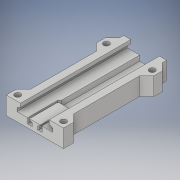
# Autodesk Inventor part: Holder_Mount
Saved by Autodesk Inventor 2019 (Build 230136000, 136)
## iProperties
Created: 2021-01-19
Part Number: Holder_Mount
Material: Generic
Document SubType Name: Modeling
Designer: zhanb
Density: 1 g/cm^3
Appearance: Default
Author: zhanb
Autodesk Inventor part; units mm, degrees
ref_plane "YZ Plane" through (0, 0, 0) normal (1, 0, 0) x (0, 1, 0)
ref_plane "XZ Plane" through (0, 0, 0) normal (0, 1, 0) x (-1, 0, 0)
ref_plane "XY Plane" through (0, 0, 0) normal (0, 0, 1) x (1, 0, 0)
sketch "Sketch1" plane through (0, 0, 0) normal (0, 1, 0) x (-1, 0, 0)
  line L0 (-25.4, 57.15) -> (25.4, 57.15)
  line L1 (25.4, 57.15) -> (25.4, -57.15)
  line L2 (25.4, -57.15) -> (-25.4, -57.15)
  line L3 (-25.4, -57.15) -> (-25.4, 57.15)
  line L4 (-25.4, 57.15) -> (25.4, -57.15) construction
  line L5 (25.4, 57.15) -> (-25.4, -57.15) construction
  point P0 (0, 0)
  dimension "d0" = 50.8
  dimension "d1" = 114.3
  constraints: 12 end point, 2 midpoint, 2 parallel, 1 horizontal, 1 perpendicular
  measures "d0" distance of L1.end L2.end
  measures "d1" distance of L2.end L0.start
extrude "Extrusion1" add sketch "Sketch1" along normal blind 15.875
ref_plane "Work Plane1" through (-25.4, 0, 31.75) normal (0, 0, 1) x (1, 0, 0)
sketch "Sketch2" plane through (-25.4, 0, 31.75) normal (0, 0, 1) x (1, 0, 0)
  line L0 (50.8, 0) -> (0, 0) construction
  line L1 (50.8, 0) -> (50.8, 15.875) construction
  line L2 (0, 15.875) -> (50.8, 15.875) construction
  line L3 (0, 0) -> (0, 15.875) construction
  line L4 (0, 15.875) -> (50.8, 15.875) construction
  line L5 (25.4, 15.875) -> (25.4, 0) construction
  line L6 (50.8, 0) -> (0, 0) construction
  line L7 (6.35, 15.875) -> (6.35, 0) construction
  circle A0 centre (25.4, 16.891) radius 5.08 construction
  line L8 (12.7, 15.875) -> (12.7, 12.7)
  line L9 (12.7, 12.7) -> (9.525, 10.8669)
  line L10 (9.525, 10.8669) -> (9.525, 7.9375)
  line L11 (9.525, 7.9375) -> (19.05, 7.9375)
  line L12 (19.05, 7.9375) -> (19.05, 3.175)
  line L13 (19.05, 3.175) -> (25.4, 3.175)
  line L14 (12.7, 15.875) -> (25.4, 15.875)
  line L15 (25.4, 15.875) -> (25.4, 3.175)
  line L16 (19.05, 7.9375) -> (25.4, 7.9375)
  line L17 (20.6375, 7.9375) -> (20.6375, 7.2665)
  line L18 (20.6375, 7.2665) -> (22.225, 6.35)
  line L19 (22.225, 6.35) -> (22.225, 3.175)
  point P0 (22.225, 4.7625)
  point P1 (19.05, 5.5562)
  dimension "d20" = 6.35
  dimension "d21" = 10.16
  dimension "d22" = 6.35
  dimension "d23" = 4.7625
  dimension "d24" = 3.175
  dimension "d25" = 3.175
  dimension "d26" = 30
  dimension "d27" = 3.175
  dimension "d28" = 3.175
  dimension "d29" = 1.016
  dimension "d45" = 1.5875
  dimension "d46" = 3.175
  dimension "d48" = 3.175
  dimension "d50" = 30
  constraints: 28 end point, 8 perpendicular, 6 midpoint, 6 point on line, 1 centre point, 1 collinear, 1 parallel, 1 vertical alignment
  measures "d20" distance between parallel lines of L3 L7
  measures "d21" diameter of A0
  measures "d22" distance between parallel lines of L5 L12
  measures "d23" distance between parallel lines of L11 L13
  measures "d24" distance between parallel lines of L7 L10
  measures "d25" distance between parallel lines of L10 L8
  measures "d26" angle of L2 L9
  measures "d27" distance between parallel lines of L0 L13
  measures "d28" distance from line of L2 L8.end
  measures "d29" distance from line of L14 A0.centre
  measures "d45" distance between parallel lines of L17 L19
  measures "d46" distance of L18.end L19.end
  measures "d48" distance between parallel lines of L5 L19
  measures "d50" angle of L16 L18
extrude "Extrusion2" cut sketch "Sketch2" against normal through all
extrude "Extrusion3" cut sketch "Sketch2" along normal through all contours L14 L15 L16 L11 L10 L9 L8 | L17 L18 L19 L13 L12 L16
sketch "Sketch7" plane through (-6.35, 3.175, -57.15) normal (0, 1, 0) x (1, 0, 0)
  line L0 (0, -114.3) -> (0, 0) construction
  line L1 (6.35, -114.3) -> (1.5875, -114.3) construction
  line L2 (6.35, -88.9) -> (6.35, -114.3) construction
  line L3 (1.5875, -88.9) -> (6.35, -88.9) construction
  line L4 (1.5875, -88.9) -> (1.5875, -114.3) construction
  line L5 (0, -87.63) -> (1.5875, -86.0425)
  line L6 (1.5875, -86.0425) -> (1.5875, 0)
  line L7 (-19.05, 0) -> (31.75, 0) projected
  line L8 (0, 0) -> (1.5875, 0)
  line L9 (0, 0) -> (0, -87.63)
  point P0 (6.35, -57.15)
  dimension "d63" = 135
  dimension "d64" = 1.5875
  dimension "d65" = 1.27
  constraints: 8 end point, 2 perpendicular, 2 point on line, 1 parallel
  measures "d63" angle of L0 L5
  measures "d64" distance between parallel lines of L0 L6
  measures "d65" vertical distance of L5.start L3.start
extrude "Extrusion6" add sketch "Sketch7" along normal up to surface (4.7625 mm away)
chamfer "Chamfer2" distance 0.762 angle 45 2 edges at (-4.7625, 7.602, 31.75) (-3.175, 4.7625, 57.15)
sketch "Sketch8" plane through (0, 15.875, 0) normal (0, 1, 0) x (1, 0, 0)
  circle A0 centre (-20.32, 26.67) radius 2.5797 construction
  line L0 (-12.7, 57.15) -> (-25.4, 57.15) construction
  line L1 (-25.4, 57.15) -> (-25.4, -57.15) construction
  line L2 (-15.875, -57.15) -> (-15.875, 57.15) construction
  line L3 (-25.4, -57.15) -> (25.4, -57.15) projected
  line L4 (-25.4, 22.86) -> (-19.05, 16.51)
  line L5 (-19.05, 16.51) -> (-19.05, -41.91)
  line L6 (-19.05, -41.91) -> (-25.4, -48.26)
  line L7 (-25.4, 22.86) -> (-25.4, -48.26)
  line L8 (-25.4, -57.15) -> (-25.4, 57.15) construction
  line L9 (-25.4, 30.48) -> (-19.05, 36.83)
  line L10 (-19.05, 36.83) -> (-19.05, 57.15)
  line L11 (-25.4, 30.48) -> (-25.4, 22.86) construction
  line L12 (-25.4, 30.48) -> (-25.4, 57.15)
  line L13 (-25.4, 57.15) -> (-19.05, 57.15)
  point P0 (0, 0)
  point P1 (-20.32, -52.07)
  point P2 (-12.7, -57.15)
  point P3 (-25.4, 26.67)
  dimension "d71" = 5.1594
  dimension "d72" = 30.48
  dimension "d73" = 5.08
  dimension "d75" = 135
  dimension "d76" = 135
  dimension "d77" = 3.175
  dimension "d89" = 34.29
  dimension "d91" = 5.08
  dimension "d92" = 8.89
  constraints: 18 end point, 4 collinear, 3 point on line, 2 midpoint, 2 vertical, 1 centre point, 1 coincident, 1 horizontal alignment, 1 perpendicular, 1 vertical alignment
  measures "d71" diameter of A0
  measures "d72" distance from line of L0 A0.centre
  measures "d73" distance from line of L1 A0.centre
  measures "d75" angle of L1 L4
  measures "d76" angle of L1 L6
  measures "d77" distance between parallel lines of L2 L5
  measures "d89" distance of L0.end L4.start
  measures "d91" distance from line of L3 point (-20.32, -52.07)
  measures "d92" distance of L1.end L6.end
hole "Hole2" at (-20.32, 15.875, -26.67) at (-20.32, 15.875, 52.07) direction (0, -1, 0) diameter 5.1562 end through all
extrude "Extrusion7" cut sketch "Sketch8" against normal through all
mirror "Mirror1" about plane through (0, 15.875, 31.75) normal (-1, 0, 0) of "Extrusion2", "Extrusion3", "Extrusion7", "Hole2", "Chamfer2", "Extrusion6"
sketch "Sketch9" plane through (0, 0, 0) normal (0, -1, 0) x (1, 0, 0)
  line L0 (19.05, -57.15) -> (19.05, -36.83) projected
  line L1 (19.05, -57.15) -> (12.7, -57.15) projected
  line L2 (-19.05, -57.15) -> (-19.05, -36.83) projected
  line L3 (19.05, -57.15) -> (-19.05, -57.15)
  line L4 (-19.05, -57.15) -> (-19.05, -40.64)
  line L5 (-19.05, -40.64) -> (19.05, -40.64)
  line L6 (19.05, -40.64) -> (19.05, -57.15)
  point P0 (0, 0)
  dimension "d93" = 16.51
  constraints: 8 end point, 2 parallel, 1 horizontal, 1 perpendicular, 1 point on line
  measures "d93" distance between parallel lines of L3 L5
extrude "Extrusion8" cut sketch "Sketch9" against normal through all
equation "\"d76\" = d75"
body "Solid1"
